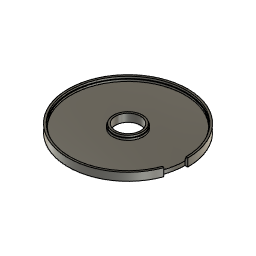
Track Base v8 (Autodesk Fusion 360 design; units mm, degrees)
Autodesk Fusion 360 part; units mm, degrees
note: some values were not read from the file. Set by a fixed rule: which sketch regions a step uses.
sketch "Sketch1" plane through (0, 0, 0) normal (1, 0, 0) x (0, 1, 0)
  line L0 (32, 0) -> (152, 0)
  line L1 (32, 0) -> (32, 29)
  line L2 (152, 0) -> (152, 29)
  line L3 (32, 29) -> (36.8, 29)
  line L4 (36.8, 29) -> (36.8, 24)
  line L5 (36.8, 24) -> (38.8, 24)
  line L6 (38.8, 24) -> (38.8, 19)
  line L7 (152, 29) -> (147.2, 29)
  line L8 (147.2, 29) -> (147.2, 24)
  line L9 (147.2, 24) -> (145.2, 24)
  line L10 (145.2, 24) -> (145.2, 19)
  line L11 (38.8, 19) -> (145.2, 19)
  dimension "d1" = 32
  dimension "d2" = 120
  dimension "d3" = 29
  dimension "d4" = 29
  dimension "d39" = 4.8
  dimension "d40" = 5
  dimension "d41" = 2
  dimension "d42" = 5
  dimension "d43" = 4.8
  dimension "d44" = 5
  dimension "d45" = 2
  dimension "d46" = 5
  constraint perpendicular L0 L1
  constraint perpendicular L0 L2
  constraint perpendicular L1 L3
  constraint perpendicular L3 L4
  constraint perpendicular L4 L5
  constraint perpendicular L5 L6
  constraint perpendicular L2 L7
  constraint perpendicular L7 L8
  constraint perpendicular L8 L9
  constraint perpendicular L9 L10
  measures "d1" distance of origin L0.start
  measures "d2" distance of L0.start L0.end
  measures "d3" distance of L0.start L1.end
  measures "d4" distance of L0.end L2.end
  measures "d39" distance of L1.end L3.end
  measures "d40" distance of L3.end L4.end
  measures "d41" distance of L4.end L5.end
  measures "d42" distance of L5.end L6.end
  measures "d43" distance of L2.end L7.end
  measures "d44" distance of L7.end L8.end
  measures "d45" distance of L8.end L9.end
  measures "d46" distance of L9.end L10.end
revolve "Revolve1" add sketch "Sketch1" angle 360 about axis through (0, 0, 1.75) along (0, 0, 1)
sketch "Sketch2" plane through (0, 0, 0) normal (0, 0, 1) x (1, 0, 0)
  line L0 (145, 0) -> (152, 0)
  line L1 (136.2554, -49.5929) -> (142.8333, -51.9871)
  arc A0 (142.8333, -51.9871) -> (152, 0) centre (0, 0) ccw
  arc A1 (136.2554, -49.5929) -> (145, 0) centre (0, 0) ccw
  dimension "d14" = 20
  dimension "d15" = 290
  dimension "d16" = 304
  constraint horizontal L0
  constraint coincident A0.centre A1.centre
  constraint concentric A0 A1
  measures "d14" angle of L0 L1
  measures "d15" diameter of A1
  measures "d16" diameter of A0
extrude "Extrude1" cut sketch "Sketch2" along normal blind 29 and the other way blind 50
extrude "Extrude2" cut 1 faces at (107.1853, 17.1871, 0) along direction (0, 0, 1) blind 5
move_body "Move1" bodies 1 to x (1, 0, 0) y (0, 1, 0) z (0, 0, 1) at (0, 0, -5)
extrude "Extrude3" cut 1 faces at (107.1853, 17.1871, 0) along direction (0, 0, 1) blind 4
